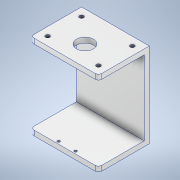
# Autodesk Inventor part: arm
Saved by Autodesk Inventor 2020 (Build 240168000, 168)
## iProperties
Created: 2020-06-25
Part Number: arm
Material: アルミニウム 6061
Document SubType Name: Modeling
Designer: haya
Density: 2.7 g/cm^3
Appearance: アルミニウム - フラット
Author: haya
Autodesk Inventor part; units mm, degrees
ref_plane "YZ Plane" through (0, 0, 0) normal (1, 0, 0) x (0, 1, 0)
ref_plane "XZ Plane" through (0, 0, 0) normal (0, 1, 0) x (-1, 0, 0)
ref_plane "XY Plane" through (0, 0, 0) normal (0, 0, 1) x (1, 0, 0)
sketch "スケッチ1" plane through (0, 0, 0) normal (0, 0, 1) x (1, 0, 0)
  line L0 (0, 0) -> (40, 0)
  line L1 (40, 0) -> (40, 50)
  line L2 (40, 50) -> (0, 50)
  line L3 (0, 50) -> (0, 0)
  dimension "d0" = 40
  dimension "d1" = 50
  constraints: 8 end point, 2 parallel, 1 horizontal, 1 perpendicular
  measures "d0" distance of L0.start L0.end
  measures "d1" distance of L2.end L0.start
extrude "押し出し1" add sketch "スケッチ1" along normal blind 3
sketch "スケッチ2" plane through (0, 0, 3) normal (0, 0, 1) x (1, 0, 0)
  line L0 (40, 50) -> (0, 50) projected
  line L1 (40, 0) -> (40, 50) projected
  line L2 (0, 50) -> (40, 50)
  line L3 (40, 50) -> (40, 47)
  line L4 (40, 47) -> (0, 47)
  line L5 (0, 47) -> (0, 50)
  line L6 (0, 50) -> (0, 0) projected
  line L7 (0, 0) -> (40, 0)
  line L8 (40, 0) -> (40, 3)
  line L9 (40, 3) -> (0, 3)
  line L10 (0, 3) -> (0, 0)
  point P0 (0, 3)
  dimension "d5" = 3
  dimension "d6" = 3
  constraints: 16 end point, 4 parallel, 2 horizontal, 2 perpendicular, 2 point on line
  measures "d5" distance between parallel lines of L0 L4
  measures "d6" distance between parallel lines of L9 L7
extrude "押し出し2" add sketch "スケッチ2" along normal blind 27 contours L1 L4 L5 L0 | L1 L7 L6 L9
sketch "スケッチ3" plane through (0, 50, 0) normal (0, 1, 0) x (1, 0, 0)
  line L0 (0, 0) -> (0, -30) projected
  line L1 (40, 0) -> (0, 0) projected
  point P0 (20, -18)
  dimension "d9" = 20
  dimension "d10" = 18
  measures "d9" distance from line of point (20, -18) L0
  measures "d10" distance from line of point (20, -18) L1
hole "穴1" at (20, 50, 18) direction (0, -1, 0) diameter 10 depth 3
sketch "スケッチ5" plane through (0, 0, 0) normal (0, -1, 0) x (1, 0, 0)
  line L0 (40, 0) -> (40, 30) projected
  line L1 (40, 15) -> (0, 15)
  line L2 (0, 3) -> (0, 30) projected
  line L3 (0, 0) -> (40, 0) projected
  line L4 (20, 0) -> (20, 30)
  line L5 (0, 30) -> (40, 30) projected
  point P0 (25, 1.5)
  point P1 (15, 1.5)
  point P2 (25, 28.5)
  point P3 (15, 28.5)
  dimension "d18" = 10
  dimension "d19" = 27
  constraints: 4 end point, 3 midpoint, 3 symmetric about line, 1 horizontal, 1 point on line
  measures "d18" distance of point (15, 1.5) point (25, 1.5)
  measures "d19" distance of point (15, 28.5) point (15, 1.5)
hole "穴2" at (25, 0, 1.5) at (15, 0, 1.5) at (25, 0, 28.5) at (15, 0, 28.5) direction (0, 1, 0) diameter 1.567 depth 4 tip angle 118 thread size "M2x0.4" class "6H" standard "ISO Metric profile"
sketch "スケッチ6" plane through (0, 50, 0) normal (0, 1, 0) x (1, 0, 0)
  line L0 (40, 0) -> (0, 0) projected
  line L1 (20, 0) -> (20, -30)
  line L2 (40, -30) -> (0, -30) projected
  line L3 (0, 0) -> (0, -30) projected
  line L4 (0, -15) -> (40, -15)
  line L5 (40, 0) -> (40, -30) projected
  point P0 (5, -5)
  point P1 (35, -5)
  point P2 (5, -25)
  point P3 (35, -25)
  dimension "d27" = 20
  dimension "d28" = 30
  constraints: 4 end point, 4 midpoint, 3 symmetric about line
  measures "d27" distance of point (5, -25) point (5, -5)
  measures "d28" distance of point (35, -5) point (5, -5)
hole "穴3" at (5, 50, 5) at (35, 50, 5) at (5, 50, 25) at (35, 50, 25) direction (0, -1, 0) diameter 2.459 depth 3 thread size "M3x0.5" class "6H" standard "ISO Metric profile"
fillet "フィレット1" radius 2 4 edges at (0, 48.5, 30) (0, 1.5, 30) (40, 48.5, 30) (40, 1.5, 30)
